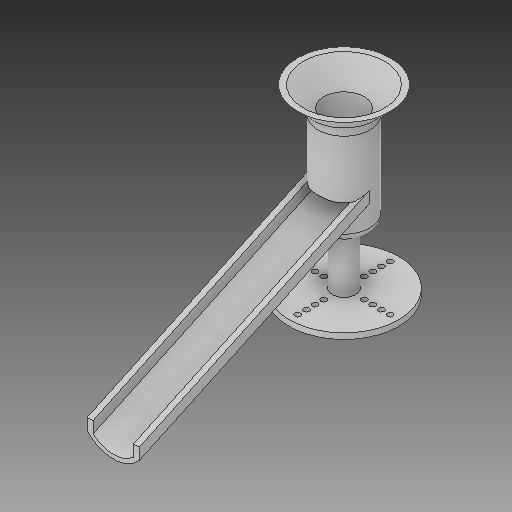
# Autodesk Inventor part: toboganANavet
Saved by Autodesk Inventor 2019 (Build 230136000, 136)
## iProperties
Created: 2021-01-18
Part Number: toboganANavet
Material: Générique
Document SubType Name: Modeling
Designer: tom.mousset
Density: 1 g/cm^3
Appearance: Par défaut
Author: tom.mousset
Autodesk Inventor part; units mm, degrees
ref_plane "YZ Plane" through (0, 0, 0) normal (1, 0, 0) x (0, 1, 0)
ref_plane "XY Plane" through (0, 0, 0) normal (0, 0, 1) x (1, 0, 0)
sketch "Esquisse2" plane through (0, 0, 0) normal (0, 0, 1) x (1, 0, 0)
  line L0 (0, 0) -> (-7, 0)
  line L1 (0, 0) -> (7, 0)
  line L2 (0, 0) -> (0, -2.6)
  arc A0 (-7, 0) -> (7, 0) centre (0, 8.1231) ccw
  line L3 (-7, 0) -> (-9, 0)
  line L4 (7, 0) -> (9, 0)
  arc A1 (-9, 0) -> (9, 0) centre (0, 8.1231) ccw
  line L5 (-9, 0) -> (-9, 4)
  line L6 (-9, 4) -> (-7, 4)
  line L7 (-7, 4) -> (-7, 0)
  line L8 (7, 0) -> (7, 4)
  line L9 (7, 4) -> (9, 4)
  line L10 (9, 4) -> (9, 0)
  line L11 (-9, 0) -> (-16.5373, 0)
  line L12 (-16.5373, 0) -> (-16.5373, -16.4452)
  line L13 (-16.5373, -16.4452) -> (24.4536, -16.4452)
  line L14 (24.4536, -16.4452) -> (24.4536, 0)
  line L15 (24.4536, 0) -> (9, 0)
  dimension "d3" = 7
  dimension "d4" = 2.6
  dimension "d5" = 2
  dimension "d6" = 4
  constraints: 32 end point, 7 perpendicular, 5 horizontal, 5 point on circle, 3 point on line, 2 centre point, 2 collinear, 2 vertical, 1 concentric, 1 parallel
  measures "d3" distance of L0.start L0.end
  measures "d4" distance of L0.start L2.end
  measures "d5" distance of L0.end L3.end
  measures "d6" distance of L3.end L5.end
sketch "Esquisse1" plane through (0, 0, 0) normal (1, 0, 0) x (0, 1, 0)
  line L0 (0, 0) -> (0, 80)
  line L1 (0, 0) -> (0, -7)
  line L2 (0, 80) -> (-134.4279, 80) construction
  line L3 (0, 0) -> (-37.3046, 80)
  line L4 (0, 0) -> (88.2702, 0) construction
  line L5 (0, 0) -> (6.9784, -14.9651)
  dimension "d0" = 80
  dimension "d1" = 7
  dimension "d2" = 115
  constraints: 12 end point, 2 horizontal, 2 vertical, 1 collinear, 1 equal length, 1 point on line
  measures "d0" distance of L0.start L0.end
  measures "d1" distance of L0.start L1.end
  measures "d2" angle of L4 L3
sweep "Balayage1" add profiles "Esquisse2" path "Esquisse1" path curves L3 contours A0 L4 A1 L3 | L3 L5 L6 L7 | L8 L9 L10 L4
sweep "Balayage2" add profiles "Esquisse2" path "Esquisse1" path curves L5 contours A0 L4 A1 L3
sketch "Esquisse3" plane through (0, 0, 0) normal (0, 1, 0) x (-1, 0, 0)
  line L0 (-7, 0) -> (-7, 80) projected
  line L1 (7, 0) -> (7, 80) projected
  arc A0 (-7, 0) -> (7, 0) centre (0, 0) ccw
  line L2 (7, 0) -> (16.2292, 0)
  line L3 (16.2292, 0) -> (12.7401, -22.6974)
  line L4 (12.7401, -22.6974) -> (-14.6528, -22.6974)
  line L5 (-14.6528, -22.6974) -> (-11.5843, 0)
  line L6 (-9, 0) -> (-7, 0) projected
  line L7 (-11.5843, 0) -> (-7, 0)
  constraints: 10 end point, 2 point on circle, 1 centre point, 1 coincident, 1 collinear, 1 horizontal, 1 parallel, 1 point on line
extrude "Extrusion1" cut sketch "Esquisse3" along normal mid plane 15
ref_plane "Plan de construction1" through (-8, 4, 0) normal (0, 1, 0) x (-1, 0, 0)
sketch "Esquisse4" plane through (-8, 4, 0) normal (0, 1, 0) x (-1, 0, 0)
  line L0 (-15, 0) -> (-15, 80) projected
  arc A0 (-15, 0) -> (-1, 0) centre (-8, 0) ccw
  line L1 (-17, 0) -> (-17, 80) projected
  line L2 (-1, 0) -> (1, 0) projected
  arc A1 (-17, 0) -> (1, 0) centre (-8, 0) ccw
  line L3 (-17, 0) -> (-15, 0)
  line L4 (-1, 0) -> (1, 0)
  constraints: 4 end point, 4 point on circle, 2 centre point, 2 coincident, 1 collinear, 1 perpendicular
extrude "Extrusion2" add sketch "Esquisse4" against normal blind 10
sketch "Esquisse6" plane through (0, 0, 0) normal (1, 0, 0) x (0, 1, 0)
  line L0 (-37.3046, 80) -> (-33.3046, 80) projected
  line L1 (-37.3046, 80) -> (31.7391, -68.0646)
  line L2 (-37.3046, 80) -> (126.0666, 80) construction
  point P0 (0, 0)
  dimension "d15" = 65
  constraints: 4 end point, 1 equal length, 1 horizontal
  measures "d15" angle of L1 L2
sweep "Balayage3" cut profiles "Esquisse2" path "Esquisse6" path curves L1 contours A1 L15 L14 L13 L12 L11
sketch "Esquisse7" plane through (-8, 4, 0) normal (0, 1, 0) x (1, 0, 0)
  line L0 (1, 0) -> (-1, 0) projected
  circle A0 centre (8, 0) radius 9
  circle A1 centre (8, 0) radius 7
  constraints: 2 coincident, 2 horizontal alignment, 4 other
extrude "Extrusion3" add sketch "Esquisse7" along normal blind 20 and the other way blind 2
sketch "Esquisse9" plane through (0, 0, 0) normal (0, 1, 0) x (-1, 0, 0)
  circle A0 centre (0, 0) radius 9
  constraints: 1 centre point, 1 coincident
extrude "Extrusion4" add sketch "Esquisse9" against normal blind 30 and the other way blind 1
sketch "Esquisse8" plane through (0, 0, 0) normal (0, 0, 1) x (1, 0, 0)
  line L0 (7, 0) -> (7, -37.3046) projected
  line L1 (7, 0) -> (7, 4)
  line L2 (7, 2) -> (7, 0) projected
  line L3 (-7, 0) -> (-7, -37.3046) projected
  line L4 (-7, 0) -> (-7, 4)
  line L5 (-7, 0) -> (-7, 24) projected
  ellipse E0 centre (0, 4) end of major axis (-9, 4) minor radius 4.1968 (7.9123, 2) -> (9, 4) ccw projected
  line L6 (-7, 4) -> (7, 4) construction
  line L7 (0, 4) -> (0, 6.6) construction
  arc A0 (7, 4) -> (-7, 4) centre (0, -4.1231) ccw
  line L8 (-7, 0) -> (7, 0)
  arc A1 (-7, 0) -> (7, 0) centre (0, 8.1231) ccw
  point P0 (0, 0)
  point P1 (7, 2.4843)
  point P2 (0, -2.6)
  dimension "d22" = 4
  dimension "d23" = 4
  dimension "d24" = 2.6
  dimension "d31" = 2.6
  constraints: 10 end point, 6 point on circle, 2 centre point, 1 collinear, 1 horizontal, 1 point on line, 1 vertical, 1 other
  measures "d22" distance of L0.start L1.end
  measures "d23" distance of L3.start L4.end
  measures "d24" distance of L7.start L7.end
  measures "d31" distance of point (0, 0) point (0, -2.6)
sweep "Balayage4" cut profiles "Esquisse8" path "Esquisse1" path curves L5 L3
extrude "Extrusion5" add sketch "Esquisse4" along normal mid plane 20
sketch "Esquisse10" plane through (0, -30, 0) normal (0, -1, 0) x (1, 0, 0)
  circle A0 centre (0, 0) radius 9 projected
  circle A1 centre (0, 0) radius 9
  circle A2 centre (0, 0) radius 4
  dimension "d34" = 8
  constraints: 2 centre point, 2 coincident
  measures "d34" diameter of A2
extrude "Extrusion6" cut sketch "Esquisse10" against normal blind 20
fillet "Congé1" radius 2.5 2 edges at (9, -10, 0) (-4, -10, 0)
sketch "Esquisse11" plane through (0, -30, 0) normal (0, -1, 0) x (1, 0, 0)
  circle A0 centre (0, 0) radius 19 construction
  circle A1 centre (0, -13) radius 1 construction
  circle A2 centre (0, -16) radius 1 construction
  circle A3 centre (0, -10) radius 1 construction
  circle A4 centre (0, -7) radius 1 construction
  arc A5 (0, -15) -> (0, -17) centre (0, -16) ccw
  arc A6 (0, -12) -> (0, -14) centre (0, -13) ccw
  arc A7 (0, -9) -> (0, -11) centre (0, -10) ccw
  arc A8 (0, -6) -> (0, -8) centre (0, -7) ccw
  line L0 (0, -19) -> (0, -17)
  line L1 (0, -15) -> (0, -14)
  line L2 (0, -12) -> (0, -11)
  line L3 (0, -9) -> (0, -8)
  circle A9 centre (0, 0) radius 6.5 projected
  line L4 (0, -6) -> (0, 0)
  line L5 (0, 0) -> (-13.435, -13.435)
  arc A10 (-13.435, -13.435) -> (0, -19) centre (0, 0) ccw
  dimension "d38" = 38
  dimension "d39" = 2
  dimension "d40" = 2
  dimension "d41" = 2
  dimension "d42" = 2
  dimension "d43" = 16
  dimension "d44" = 13
  dimension "d45" = 10
  dimension "d46" = 7
  dimension "d47" = 45
  constraints: 20 point on circle, 12 end point, 10 centre point, 6 coincident, 4 concentric, 3 collinear, 2 vertical
  measures "d38" diameter of A0
  measures "d39" diameter of A1
  measures "d40" diameter of A2
  measures "d41" diameter of A3
  measures "d42" diameter of A4
  measures "d43" distance of point (0, 0) A2.centre
  measures "d44" distance of point (0, 0) A1.centre
  measures "d45" distance of point (0, 0) A3.centre
  measures "d46" distance of point (0, 0) A4.centre
  measures "d47" angle of L5 L4
extrude "Extrusion7" add sketch "Esquisse11" along normal blind 2 contours A5 L0 A10 L5 A9 A8 L3 A7 L2 A6 L1 | L5 L4 A8 A9 picked at (-0.8189, -4.0472)
mirror "Symétrie1" about plane through (0, 0, 0) normal (1, 0, 0) of "Extrusion7"
pattern_circular "Réseau circulaire1" count 4 over 360 about axis through (0, -10, 0) along (0, 1, 0) of "Extrusion7", "Symétrie1"
sketch "Esquisse12" plane through (0, 0, 0) normal (1, 0, 0) x (0, 1, 0)
  line L0 (24, -9) -> (34, -9) construction
  line L1 (24, 7) -> (24, -7) projected
  line L2 (24, -9) -> (24, -7)
  line L3 (24, -7) -> (31.0711, -14.0711)
  line L4 (24, -7) -> (34, -7) construction
  line L5 (31.0711, -14.0711) -> (31.0711, -16.0711)
  line L6 (31.0711, -16.0711) -> (24, -9)
  line L7 (-6.8, 0) -> (40.8, 0) projected
  point P0 (0, 0)
  dimension "d56" = 10
  dimension "d57" = 45
  dimension "d58" = 2
  constraints: 12 end point, 2 horizontal, 2 vertical, 1 equal length
  measures "d56" distance of L1.end L3.end
  measures "d57" angle of L3 L4
  measures "d58" distance of L3.end L5.end
revolve "Révolution1" add sketch "Esquisse12" angle 360 about axis through (0, -10, 0) along (0, 1, 0)
fillet "Congé2" radius 5 1 edges at (6.364, 24, -6.364)
